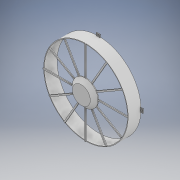
# Autodesk Inventor part: Ventilator
Saved by Autodesk Inventor 2021 (Build 250183000, 183)
## iProperties
Created: 2021-09-01
Part Number: Ventilator
Material: Generisch
Document SubType Name: Modeling
Designer: lukas
Density: 1 g/cm^3
Appearance: Vorgabe
Author: lukas
Autodesk Inventor part; units mm, degrees
ref_plane "YZ Plane" through (0, 0, 0) normal (1, 0, 0) x (0, 1, 0)
ref_plane "XZ Plane" through (0, 0, 0) normal (0, 1, 0) x (-1, 0, 0)
ref_plane "XY Plane" through (0, 0, 0) normal (0, 0, 1) x (1, 0, 0)
sketch "Skizze1" plane through (0, 0, 0) normal (0, 0, 1) x (1, 0, 0)
  line L0 (-245, 0) -> (245, 0) projected
  line L1 (0, -245) -> (0, 245) projected
  line L2 (175, 7.5) -> (175, -7.5)
  line L3 (-175, -7.5) -> (-175, 7.5)
  line L4 (-7.5, 175) -> (7.5, 175)
  line L5 (7.5, -175) -> (-7.5, -175)
  circle A0 centre (0, 170) radius 2.5
  circle A1 centre (0, -170) radius 2.5
  circle A2 centre (-170, 0) radius 2.5
  circle A3 centre (170, 0) radius 2.5
  circle A4 centre (0, 0) radius 165
  line L6 (7.5, 175) -> (7.5, 164.8295)
  line L7 (-7.5, 164.8295) -> (-7.5, 175)
  line L8 (-175, 7.5) -> (-164.8295, 7.5)
  line L9 (-164.8295, -7.5) -> (-175, -7.5)
  line L10 (175, -7.5) -> (164.8295, -7.5)
  line L11 (164.8295, 7.5) -> (175, 7.5)
  line L12 (7.5, -164.8295) -> (7.5, -175)
  line L13 (-7.5, -175) -> (-7.5, -164.8295)
  circle A5 centre (0, 0) radius 162.5
  dimension "d12" = 330
  dimension "d2" = 350
  dimension "d3" = 350
  dimension "d4" = 5
  dimension "d5" = 5
  dimension "d6" = 5
  dimension "d7" = 5
  dimension "d8" = 5
  dimension "d9" = 5
  dimension "d10" = 5
  dimension "d11" = 5
  dimension "d13" = 325
  constraints: 24 end point, 10 parallel, 6 coincident, 5 centre point, 4 perpendicular, 4 point on line, 3 horizontal, 12 other
  measures "d2" distance between parallel lines of L2 L3
  measures "d3" distance from line of L4.end L5
  measures "d4" distance from line of L4 point (0, 170)
  measures "d5" diameter of A0
  measures "d6" distance from line of point (0, -170) L5
  measures "d7" diameter of A1
  measures "d8" distance from line of point (-170, 0) L3
  measures "d9" distance from line of L2 point (170, 0)
  measures "d10" diameter of A2
  measures "d11" diameter of A3
  measures "d13" diameter of A5
extrude "Extrusion1" add sketch "Skizze1" along normal blind 3 contours A4 L11 L2 L0 A3 | L0 A3 L2 L10 A4 | A4 L7 L4 L1 A0 | L1 A0 L4 L6 A4 | A4 L12 L5 L1 A1 | L1 A1 L5 L13 A4 | A4 L9 L3 L0 A2 | L0 A2 L3 L8 A4
sketch "Skizze2" plane through (0, 0, 0) normal (0, 0, 1) x (1, 0, 0)
  line L0 (-231, 0) -> (231, 0) projected
  line L1 (0, -231) -> (0, 231) projected
  circle A0 centre (0, 0) radius 165
  circle A1 centre (0, 0) radius 162.5
  dimension "d16" = 330
  dimension "d17" = 325
  constraints: 2 centre point, 2 coincident
  measures "d16" diameter of A0
  measures "d17" diameter of A1
extrude "Extrusion2" add sketch "Skizze2" along normal blind 50
sketch "Skizze3" plane through (0, 0, 50) normal (0, 0, 1) x (1, 0, 0)
  circle A0 centre (0, 0) radius 162.5
  dimension "d20" = 325
  constraints: 1 centre point, 1 coincident
  measures "d20" diameter of A0
extrude "Extrusion3" cut sketch "Skizze3" against normal blind 50
sketch "Skizze5" plane through (0, 0, 50) normal (0, 0, 1) x (1, 0, 0)
  line L0 (-249.0675, 0) -> (269.4048, 0) projected
  line L1 (0, -269.4048) -> (0, 249.0675) projected
  line L2 (-2.5, 165) -> (2.5, 165)
  line L3 (2.5, 165) -> (2.5, -165)
  line L4 (2.5, -165) -> (-2.5, -165)
  line L5 (-2.5, -165) -> (-2.5, 165)
  line L6 (-165, 2.5) -> (165, 2.5)
  line L7 (165, 2.5) -> (165, -2.5)
  line L8 (165, -2.5) -> (-165, -2.5)
  line L9 (-165, -2.5) -> (-165, 2.5)
  circle A0 centre (0, 0) radius 165 projected
  circle A1 centre (0, 0) radius 162.5 projected
  line L10 (-80.3255, 144.1278) -> (0, 5)
  line L11 (-84.6556, 141.6278) -> (-6.8301, 6.8301)
  line L12 (-6.8301, 6.8301) -> (-141.6278, 84.6556)
  line L13 (-9.3301, 2.5) -> (-144.1278, 80.3255)
  line L14 (0, 5) -> (80.3255, 144.1278)
  line L15 (6.8301, 6.8301) -> (84.6556, 141.6278)
  line L16 (9.3301, 2.5) -> (144.1278, 80.3255)
  line L17 (6.8301, 6.8301) -> (141.6278, 84.6556)
  line L18 (-144.1278, -80.3255) -> (-9.3301, -2.5)
  line L19 (-141.6278, -84.6556) -> (-6.8301, -6.8301)
  line L20 (-80.3255, -144.1278) -> (-2.5, -9.3301)
  line L21 (-84.6556, -141.6278) -> (-6.8301, -6.8301)
  arc A2 (7.5, -164.8295) -> (164.8295, -7.5) centre (0, 0) ccw projected
  line L22 (2.5, -9.3301) -> (80.3255, -144.1278)
  line L23 (6.8301, -6.8301) -> (141.6278, -84.6556)
  line L24 (144.1278, -80.3255) -> (9.3301, -2.5)
  line L25 (84.6556, -141.6278) -> (6.8301, -6.8301)
  line L26 (141.6278, -84.6556) -> (144.1278, -80.3255)
  line L27 (141.6278, 84.6556) -> (144.1278, 80.3255)
  line L28 (80.3255, 144.1278) -> (84.6556, 141.6278)
  line L29 (-84.6556, 141.6278) -> (-80.3255, 144.1278)
  line L30 (-144.1278, 80.3255) -> (-141.6278, 84.6556)
  line L31 (-141.6278, -84.6556) -> (-144.1278, -80.3255)
  line L32 (-80.3255, -144.1278) -> (-84.6556, -141.6278)
  point P0 (-142.8942, 82.5)
  point P1 (79.0753, -141.9625)
  point P2 (83.4054, -139.4625)
  point P3 (139.4625, -83.4054)
  point P4 (141.9625, -79.0753)
  point P5 (141.9625, 79.0753)
  point P6 (139.4625, 83.4054)
  point P7 (83.4054, 139.4625)
  point P8 (79.0753, 141.9625)
  point P9 (2.5, 9.3301)
  point P10 (-2.5, 9.3301)
  point P11 (-79.0753, 141.9625)
  point P12 (-83.4054, 139.4625)
  point P13 (-139.4625, 83.4054)
  point P14 (-141.9625, 79.0753)
  point P15 (-141.9625, -79.0753)
  point P16 (-139.4625, -83.4054)
  point P17 (-83.4054, -139.4625)
  point P18 (-79.0753, -141.9625)
  dimension "d23" = 5
  dimension "d24" = 5
  dimension "d25" = 330
  dimension "d26" = 330
  dimension "d30" = 5
  dimension "d34" = 5
  dimension "d37" = 5
  dimension "d38" = 5
  dimension "d43" = 5
  dimension "d44" = 5
  dimension "d46" = 5
  constraints: 62 end point, 9 parallel, 7 perpendicular, 7 point on line, 4 point on circle, 2 horizontal, 18 other
  measures "d23" distance between parallel lines of L6 L8
  measures "d24" distance between parallel lines of L3 L5
  measures "d25" distance between parallel lines of L2 L4
  measures "d26" distance between parallel lines of L9 L7
  measures "d30" distance between parallel lines of L10 L11
  measures "d34" distance between parallel lines of L12 L13
  measures "d37" distance between parallel lines of L15 L14
  measures "d38" distance between parallel lines of L17 L16
  measures "d43" distance between parallel lines of L19 L18
  measures "d44" distance between parallel lines of L20 L21
  measures "d46" distance between parallel lines of L24 L23
extrude "Extrusion4" add sketch "Skizze5" along normal blind 3 contours A1 L6 A0 L0 | A1 L8 L3 L0 | L0 L3 L6 A1 | L0 A0 L8 A1 | A0 L6 L7 | L7 L8 A0 | L3 L8 L1 L0 | L0 L1 L6 L3 | L1 L8 L5 L0 | L0 L5 L6 L1 | L6 L1 L14 L3 | L3 L14 A1 L15 L17 L16 L6 | L8 L24 A1 L23 L25 L22 L3 | L3 A1 L1 L8 | L5 L8 A1 L0 | L0 A1 L6 L5 | L1 A1 L5 L8 | L6 L5 L10 L1 | L14 L1 A1 L3 | A1 L8 A0 L0 | L0 A0 L6 A1 | L5 L20 A1 L21 L19 L18 L8 | L6 L13 A1 L12 L11 L10 L5 | A1 L3 A0 L1 | L1 A0 L5 A1 | L10 L5 A1 L1 | A1 L1 A0 L3 | A0 L8 L9 | L9 L6 A0 | A0 L3 L4 | L4 L5 A0 | A1 L5 A0 L1 | A0 L2 L3 | A0 L5 L2
sketch "Skizze6" plane through (0, 0, 53) normal (0, 0, 1) x (1, 0, 0)
  circle A0 centre (0, 0) radius 50
  dimension "d49" = 100
  constraints: 1 centre point, 1 coincident
  measures "d49" diameter of A0
extrude "Extrusion5" add sketch "Skizze6" along normal blind 15 draft -45 and the other way blind 3
sketch "Skizze7" plane through (0, 0, 50) normal (0, 0, -1) x (-1, 0, 0)
  circle A0 centre (0, 0) radius 5
  dimension "d54" = 10
  constraints: 1 centre point, 1 coincident
  measures "d54" diameter of A0
extrude "Extrusion6" cut sketch "Skizze7" against normal blind 10
